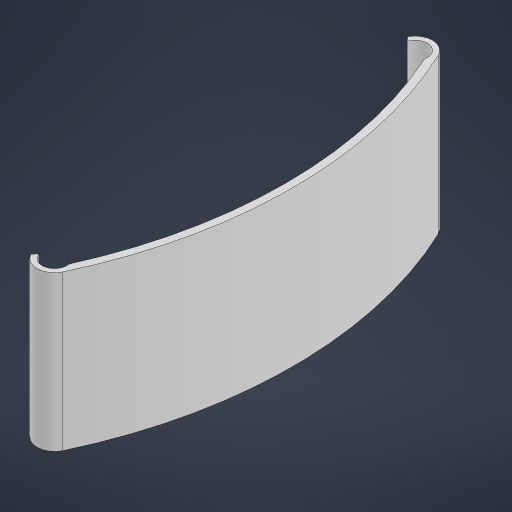
# Autodesk Inventor part: Machine_Cover
Saved by Autodesk Inventor 2024.2 (Build 282272000, 272)
## iProperties
Created: 2024-02-29
Part Number: Machine_Cover
Material: 一般
Document SubType Name: Modeling
Designer: Hanaoka
Density: 1 g/cm^3
Appearance: 既定
Author: Hanaoka
Autodesk Inventor part; units mm, degrees
ref_plane "YZ Plane" through (0, 0, 0) normal (1, 0, 0) x (0, 1, 0)
ref_plane "XZ Plane" through (0, 0, 0) normal (0, 1, 0) x (-1, 0, 0)
ref_plane "XY Plane" through (0, 0, 0) normal (0, 0, 1) x (1, 0, 0)
sketch "スケッチ1" plane through (0, 0, 0) normal (0, 1, 0) x (-1, 0, 0)
  arc A0 (8.4334, 37.592) -> (8.4334, -37.592) centre (88, 0) ccw
  arc A1 (8.5926, 34.3032) -> (8.5926, -34.3032) centre (88, 0) ccw
  line L0 (0, -123.2) -> (0, 123.2) construction
  line L1 (211.2, 0) -> (-35.2, 0) construction
  line L2 (88, 0) -> (38.8561, -49.1439)
  line L3 (88, 0) -> (38.8561, 49.1439)
  circle A2 centre (88, 0) radius 88 construction
  line L4 (38.8561, -49.1439) -> (21.1784, -31.4663) construction
  line L5 (21.1784, -31.4663) -> (10.6608, -41.9839) construction
  line L6 (38.8561, 49.1439) -> (21.1784, 31.4663) construction
  line L7 (21.1784, 31.4663) -> (10.6608, 41.9839) construction
  circle A3 centre (11.598, 36.0969) radius 3.5
  circle A4 centre (11.598, 36.0969) radius 2.5
  circle A5 centre (11.598, -36.0969) radius 3.5
  circle A6 centre (11.598, -36.0969) radius 2.5
  arc A7 (14.7014, 37.7152) -> (12.2579, 32.6597) centre (21.1784, 31.4663) ccw
  arc A8 (12.2579, -32.6597) -> (14.7014, -37.7152) centre (21.1784, -31.4663) ccw
  arc A9 (9.1534, 35.5734) -> (10.45, -38.3177) centre (88, 0) ccw
  point P0 (0, 0)
  point P1 (12.4744, 33.7556)
  point P2 (13.9772, 36.8646)
  point P3 (8.4334, -37.592)
  point P4 (14.7014, -37.7152)
  point P5 (13.9772, -36.8646)
  point P6 (12.4744, -33.7556)
  point P7 (12.2579, -32.6597)
  point P8 (8.5926, -34.3032)
  point P9 (8.5926, 34.3032)
  point P10 (9.1534, -35.5734)
  point P11 (8.5926, -34.3032)
  dimension "d6" = 5
  dimension "d0" = 88
  dimension "d2" = 86.5
  dimension "d3" = 69.5
  dimension "d4" = 176
  dimension "d5" = 25
  dimension "d7" = 7
  dimension "d8" = 9
  constraints: 16 point on circle, 12 end point, 8 centre point, 8 symmetric about line, 6 coincident, 6 perpendicular, 3 tangent, 1 concentric, 1 horizontal, 1 midpoint, 8 other
  measures "d0" radius of A0
  measures "d2" radius of A1
  measures "d3" distance of L2.start L3.end
  measures "d4" diameter of A2
  measures "d5" distance of L3.end L6.end
  measures "d7" diameter of A3
  measures "d8" radius of A7
extrude "押し出し1" add sketch "スケッチ1" along normal blind 31 contours A3 A1 A5 A0 | A3 A7 A4 A9 | A5 A9 A6 A8 picked at (10.6807, 39.1053) picked at (8.9829, -37.8462)
